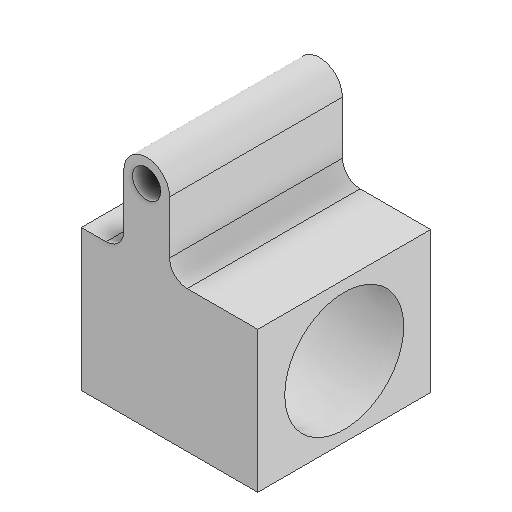
# Autodesk Inventor part: PlacaExcavacion2
Saved by Autodesk Inventor 2025.2 (Build 292293000, 293)
## iProperties
Created: 2025-08-05
Part Number: PlacaExcavacion2
Material: Generic
Document SubType Name: Modeling
Designer: Compa
Density: 1 g/cm^3
Appearance: Default
Author: Compa
Autodesk Inventor part; units mm, degrees
ref_plane "YZ Plane" through (0, 0, 0) normal (1, 0, 0) x (0, 1, 0)
ref_plane "XZ Plane" through (0, 0, 0) normal (0, 1, 0) x (-1, 0, 0)
ref_plane "XY Plane" through (0, 0, 0) normal (0, 0, 1) x (1, 0, 0)
sketch "Sketch1" plane through (0, 0, 0) normal (0, 0, 1) x (1, 0, 0)
  line L0 (0, 0) -> (0, 20)
  circle A0 centre (6.5, 20) radius 6.5
  circle A1 centre (6.5, 20) radius 4
  line L1 (13, 20) -> (13, 0)
  line L2 (13, 0) -> (0, 0)
  dimension "d0" = 20
  constraints: 6 end point, 2 vertical, 1 centre point, 1 coincident, 1 perpendicular, 3 other
  measures "d0" distance of L0.start L0.end
extrude "Extrusion1" add sketch "Sketch1" along normal mid plane 49
sketch "Sketch2" plane through (13, 0, 24.5) normal (1, 0, 0) x (0, 0, -1)
  line L0 (49, 0) -> (0, 0) projected
  line L1 (0, 0) -> (0, -40)
  line L2 (0, -40) -> (49, -40)
  line L3 (49, -40) -> (49, 0)
  line L4 (0, -40) -> (24.5, -40)
  line L5 (24.5, -40) -> (24.5, -20)
  circle A0 centre (24.5, -20) radius 20
  circle A1 centre (24.5, -20) radius 16.85
  point P0 (24.5, 0)
  dimension "d11" = 40
  dimension "d12" = 24.5
  dimension "d13" = 20
  dimension "d14" = 33.7
  constraints: 10 end point, 3 perpendicular, 2 coincident, 1 centre point, 1 midpoint, 1 vertical, 1 vertical alignment, 2 other
  measures "d11" distance of L0.end L1.end
  measures "d12" distance of L1.end L4.end
  measures "d13" distance of L4.end L5.end
  measures "d14" diameter of A1
extrude "Extrusion2" add sketch "Sketch2" along normal mid plane 50
fillet "Fillet1" radius 5 1 edges at (13, 0, 0)
fillet "Fillet2" radius 5 1 edges at (0, 0, 0)
body "Solid1"
